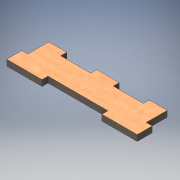
# Autodesk Inventor part: batN
Saved by Autodesk Inventor 2019 (Build 230136000, 136)
## iProperties
Created: 2020-12-06
Part Number: batN
Material: Дерево (береза)
Document SubType Name: Modeling
Designer: Professional
Density: 0.55 g/cm^3
Appearance: Береза — натуральный — полированный
Author: Professional
Autodesk Inventor part; units mm, degrees
ref_plane "YZ Plane" through (0, 0, 0) normal (1, 0, 0) x (0, 1, 0)
ref_plane "XZ Plane" through (0, 0, 0) normal (0, 1, 0) x (-1, 0, 0)
ref_plane "XY Plane" through (0, 0, 0) normal (0, 0, 1) x (1, 0, 0)
sketch "Эскиз1" plane through (0, 0, 0) normal (0, 1, 0) x (-1, 0, 0)
  line L0 (43.5, 4) -> (43.5, -6)
  line L1 (43.5, -6) -> (39.5, -6)
  line L2 (39.5, -6) -> (39.5, -20)
  line L3 (39.5, -20) -> (27.5, -20)
  line L4 (27.5, -20) -> (27.5, -16)
  line L5 (27.5, -16) -> (7.5, -16)
  line L6 (7.5, -16) -> (7.5, -20)
  line L7 (7.5, -20) -> (0, -20)
  line L8 (0, -20) -> (0, 0)
  line L9 (-43.5, 4) -> (-43.5, -6)
  line L10 (-43.5, -6) -> (-39.5, -6)
  line L11 (-39.5, -6) -> (-39.5, -20)
  line L12 (-39.5, -20) -> (-27.5, -20)
  line L13 (-27.5, -20) -> (-27.5, -16)
  line L14 (-27.5, -16) -> (-7.5, -16)
  line L15 (-7.5, -16) -> (-7.5, -20)
  line L16 (-7.5, -20) -> (0, -20)
  line L17 (43.5, 4) -> (20, 4)
  line L18 (20, 4) -> (20, 0)
  line L19 (20, 0) -> (0, 0)
  line L20 (-43.5, 4) -> (-20, 4)
  line L21 (-20, 4) -> (-20, 0)
  line L22 (-20, 0) -> (0, 0)
  dimension "d0" = 12
  dimension "d1" = 20
  dimension "d2" = 15
  dimension "d3" = 4
  dimension "d4" = 14
  dimension "d5" = 10
  dimension "d8" = 40
  constraints: 46 end point, 10 symmetric about line, 9 perpendicular, 4 point on line, 2 equal length, 1 horizontal, 1 vertical
  measures "d0" distance of L2.end L3.end
  measures "d1" distance of L4.end L5.end
  measures "d2" diameter of L6 L8
  measures "d3" distance of L3.end L4.end
  measures "d4" distance of L1.end L2.end
  measures "d5" distance of L0.start L0.end
  measures "d8" diameter of L18 L8
extrude "Выдавливание1" add sketch "Эскиз1" along normal blind 4
